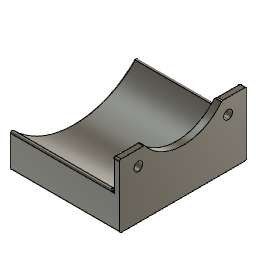
ME0907 test cradle (Autodesk Fusion 360 design; units mm, degrees)
Autodesk Fusion 360 part; units mm, degrees
note: some values were not read from the file. Set by a fixed rule: which sketch regions a step uses.
sketch "Sketch1" plane through (0, 0, 0) normal (0, 0, 1) x (1, 0, 0)
  line L0 (65, -75) -> (-65, -75)
  line L1 (-65, -75) -> (-65, 75)
  line L2 (-65, 75) -> (65, 75)
  line L3 (65, 75) -> (65, -75)
  line L4 (65, -75) -> (-65, 75) construction
  line L5 (-65, -75) -> (65, 75) construction
  dimension "d1" = 130
  dimension "d2" = 150
  constraint horizontal L0
  constraint perpendicular L0 L1
  constraint parallel L0 L2
  constraint parallel L1 L3
  constraint coincident L4 origin
  constraint coincident L5 origin
  measures "d1" distance of L1.end L2.end
  measures "d2" distance of L0.end L1.end
extrude "Extrude1" add sketch "Sketch1" along normal blind 75
sketch "Sketch2" plane through (65, 0, 0) normal (1, 0, 0) x (0, 1, 0)
  line L0 (-75, 0) -> (75, 0)
  line L1 (75, 0) -> (75, 75)
  line L2 (75, 75) -> (-75, 75)
  line L3 (-75, 75) -> (-75, 0)
  line L4 (0, 0) -> (0, 10)
  line L5 (0, 10) -> (0, 110)
  circle A0 centre (0, 110) radius 100.5
  circle A1 centre (0, 110) radius 74.615
  line L6 (0, 110) -> (52.7608, 57.2392)
  line L7 (0, 110) -> (74.615, 110) construction
  line L8 (0, 110) -> (-52.7608, 57.2392)
  line L9 (0, 110) -> (74.615, 110) construction
  circle A2 centre (52.7608, 57.2392) radius 5.2
  circle A3 centre (-52.7608, 57.2392) radius 5.2
  circle A4 centre (0, 110) radius 57.5
  dimension "d5" = 10
  dimension "d6" = 100
  dimension "d7" = 201
  dimension "d8" = 149.23
  dimension "d9" = 45
  dimension "d10" = 135
  dimension "d11" = 10.4
  dimension "d12" = 10.4
  dimension "d13" = 115
  constraint coincident L4.start origin
  constraint perpendicular L0 L4
  constraint perpendicular L2 L5
  constraint coincident L5.end A0.centre
  constraint horizontal L7
  constraint horizontal L9
  constraint coincident L6.end A2.centre
  constraint coincident L8.end A3.centre
  constraint concentric A0 A4
  measures "d5" distance of L4.start L4.end
  measures "d6" distance of L4.end L5.end
  measures "d7" diameter of A0
  measures "d8" diameter of A1
  measures "d9" angle of L6 L7
  measures "d10" angle of L8 L9
  measures "d11" diameter of A2
  measures "d12" diameter of A3
  measures "d13" diameter of A4
extrude "Extrude2" cut sketch "Sketch2" against normal blind 130 contours L2 L6 L8 A4 | L2 L8 A4 | L2 L5 L8 A4 | L2 L5 L6 A4 | L2 L5 L8 | L2 L6 A4 | L2 L5 L6
extrude "Extrude3" cut sketch "Sketch2" against normal blind 122 from surface at -8 contours L2 L3 L4 L5 A0 A1 A3 | L1 L2 L4 L5 A0 A1 A2 | L2 A1 L8 A3 A4 | L5 A1 L8 A3 A4 | L5 A1 L6 A2 A4 | A1 L8 A3 | A1 A3 | L2 A1 L6 A2 A4 | A1 L8 A3 | A1 L6 A2 | A1 A2 | A1 L6 A2
extrude "Extrude4" cut sketch "Sketch2" against normal blind 10 contours A1 L8 A3 | A1 A3 | A1 L8 A3 | A1 L6 A2 | A1 A2 | A1 L6 A2
fillet "Fillet1" radius 2 16 edges at (-65, 75, 21.5513) (-65, -75, 21.5513) (0, -75, 0) (0, 75, 0) (-4, -75, 43.1027) (-4, 75, 43.1027) (57, 60.3104, 75) (57, 75, 59.0513) (57, -75, 59.0513) (57, -60.3104, 75) (-65, 0, 9.5) (-65, 0, 0) (61, -75, 75) (61, 75, 75) (61, 45.6207, 75) (61, -45.6207, 75)
fillet "Fillet2" radius 3 5 edges at (57.5858, -74.4142, 39.4611) (57, -72.228, 39.8919) (57, 0, 9.5) (57, 72.228, 39.8919) (57.5858, 74.4142, 39.4611)
sketch "Sketch3" plane through (0, 0, 0) normal (0, 0, -1) x (1, 0, 0)
  line L0 (-63, -73) -> (65, -73)
  line L1 (65, -73) -> (65, 73)
  line L2 (65, 73) -> (-63, 73)
  line L3 (-63, 73) -> (-63, -73)
  line L4 (-63, 73) -> (-43, 73)
  line L5 (-43, 73) -> (-43, 53)
  line L6 (-38.6582, 45.5068) -> (-34.3398, 53.0135)
  line L7 (-34.3398, 53.0135) -> (-38.6816, 60.5067)
  line L8 (-38.6816, 60.5067) -> (-47.3418, 60.4932)
  line L9 (-47.3418, 60.4932) -> (-51.6602, 52.9865)
  line L10 (-51.6602, 52.9865) -> (-47.3184, 45.4933)
  line L11 (-47.3184, 45.4933) -> (-38.6582, 45.5068)
  line L12 (65, 73) -> (45, 73)
  line L13 (45, 73) -> (45, 53)
  line L14 (49.3301, 45.5) -> (53.6603, 53)
  line L15 (53.6603, 53) -> (49.3301, 60.5)
  line L16 (49.3301, 60.5) -> (40.6699, 60.5)
  line L17 (40.6699, 60.5) -> (36.3397, 53)
  line L18 (36.3397, 53) -> (40.6699, 45.5)
  line L19 (40.6699, 45.5) -> (49.3301, 45.5)
  line L20 (-63, -73) -> (-63, -53)
  line L21 (-63, -53) -> (-43, -53)
  line L22 (-38.6699, -60.5) -> (-34.3397, -53)
  line L23 (-34.3397, -53) -> (-38.6699, -45.5)
  line L24 (-38.6699, -45.5) -> (-47.3301, -45.5)
  line L25 (-47.3301, -45.5) -> (-51.6603, -53)
  line L26 (-51.6603, -53) -> (-47.3301, -60.5)
  line L27 (-47.3301, -60.5) -> (-38.6699, -60.5)
  line L28 (65, -73) -> (45, -73)
  line L29 (45, -73) -> (45, -53)
  line L30 (49.3301, -60.5) -> (53.6603, -53)
  line L31 (53.6603, -53) -> (49.3301, -45.5)
  line L32 (49.3301, -45.5) -> (40.6699, -45.5)
  line L33 (40.6699, -45.5) -> (36.3397, -53)
  line L34 (36.3397, -53) -> (40.6699, -60.5)
  line L35 (40.6699, -60.5) -> (49.3301, -60.5)
  point P0 (-43, 53)
  point P1 (45, 53)
  point P2 (-43, -53)
  point P3 (45, -53)
  dimension "d45" = 20
  dimension "d46" = 20
  dimension "d47" = 7.5
  dimension "d48" = 20
  dimension "d49" = 20
  dimension "d50" = 7.5
  dimension "d51" = 20
  dimension "d52" = 20
  dimension "d53" = 7.5
  dimension "d54" = 20
  dimension "d55" = 20
  dimension "d56" = 7.5
  constraint coincident L2.end L3.start
  constraint coincident L2 L4.end
  constraint perpendicular L4 L5
  constraint coincident P0 L5.end
  constraint coincident L1.end L2.start
  constraint perpendicular L1 L12
  constraint perpendicular L12 L13
  constraint coincident P1 L13.end
  constraint coincident L0.start L3.end
  constraint perpendicular L0 L20
  constraint perpendicular L3 L21
  constraint coincident P2 L21.end
  constraint coincident L0.end L1.start
  constraint perpendicular L1 L28
  constraint perpendicular L28 L29
  constraint coincident P3 L29.end
  measures "d45" distance of L2.end L4.end
  measures "d46" distance of L4.end P0
  measures "d47" distance of P0 L11
  measures "d48" distance of L1.end L12.end
  measures "d49" distance of L12.end P1
  measures "d50" distance of P1 L19
  measures "d51" distance of L0.start L20.end
  measures "d52" distance of L20.end P2
  measures "d53" distance of P2 L27
  measures "d56" distance of P3 L35
extrude "Extrude5" cut sketch "Sketch3" against normal blind 5 contours L6 L7 L8 L9 L10 L11 | L14 L15 L16 L17 L18 L19 | L22 L23 L24 L25 L26 L27 | L30 L31 L32 L33 L34 L35
